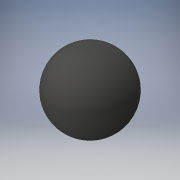
# Autodesk Inventor part: balle
Saved by Autodesk Inventor 2016 (Build 200138000, 138)
## iProperties
Created: 2016-01-25
Part Number: balle
Material: Generic
Document SubType Name: Modeling
Designer: ares-b02
Density: 1 g/cm^3
Appearance: Rubber - Black
Author: ares-b02
Autodesk Inventor part; units mm, degrees
ref_plane "YZ Plane" through (0, 0, 0) normal (1, 0, 0) x (0, 1, 0)
ref_plane "XZ Plane" through (0, 0, 0) normal (0, 1, 0) x (-1, 0, 0)
ref_plane "XY Plane" through (0, 0, 0) normal (0, 0, 1) x (1, 0, 0)
sketch "Sketch1" plane through (0, 0, 0) normal (0, 0, 1) x (1, 0, 0)
  arc A0 (-21.0728, 136.3924) -> (-21.0728, -117.6076) centre (-21.0728, 9.3924) ccw
  line L0 (-21.0728, 136.3924) -> (-21.0728, -117.6076)
  dimension "d1" = 127
  dimension "d3" = 254
  constraints: 2 end point, 2 point on circle, 1 centre point, 1 vertical
  measures "d1" radius of A0
  measures "d3" distance of L0.start L0.end
revolve "Revolution1" add sketch "Sketch1" angle 360 about axis through (-21.0728, 136.3924, 0) along (0, -1, 0)
body "Solid1"
